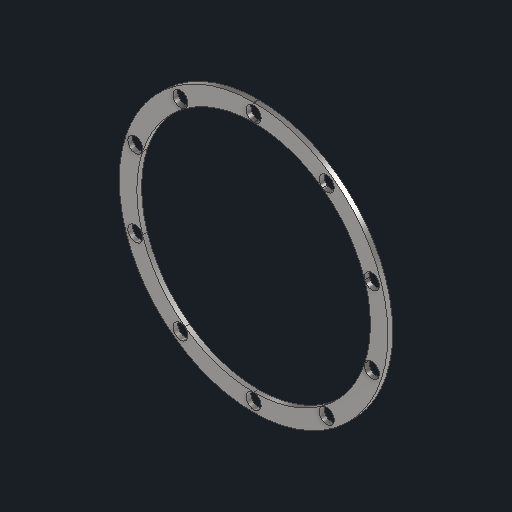
# Autodesk Inventor part: bracket 1
Saved by Autodesk Inventor 2023 (Build 270158000, 158)
## iProperties
Created: 2022-07-21
Part Number: bracket 1
Material: Stainless Steel
Document SubType Name: Modeling
Designer: station
Density: 8 g/cm^3
Appearance: Semi-Polished
Mass: 114.58 g
Surface Area: 134.314 cm^2
Volume: 14.3225 cm^3
Author: station
Autodesk Inventor part; units mm, degrees
ref_plane "YZ Plane" through (0, 0, 0) normal (1, 0, 0) x (0, 1, 0)
ref_plane "XZ Plane" through (0, 0, 0) normal (0, 1, 0) x (-1, 0, 0)
ref_plane "XY Plane" through (0, 0, 0) normal (0, 0, 1) x (1, 0, 0)
sketch "Sketch1" plane through (0, 0, 0) normal (0, 0, 1) x (1, 0, 0)
  point P0 (0, 0)
sketch "Sketch2" plane through (0, 0, 0) normal (0, 0, 1) x (1, 0, 0)
  circle A0 centre (0, 0) radius 73.505
  circle A1 centre (0, 0) radius 84.555
  line L0 (0, 0) -> (0, 267.2238)
  line L1 (0, 73.505) -> (0, 78.2675)
  circle A2 centre (0, 78.2675) radius 4.7625
  circle A3 centre (-46.0045, 63.3197) radius 4.7625
  circle A4 centre (-74.4368, 24.186) radius 4.7625
  circle A5 centre (-74.4368, -24.186) radius 4.7625
  circle A6 centre (-46.0045, -63.3197) radius 4.7625
  circle A7 centre (0, -78.2675) radius 4.7625
  circle A8 centre (46.0045, -63.3197) radius 4.7625
  circle A9 centre (74.4368, -24.186) radius 4.7625
  circle A10 centre (74.4368, 24.186) radius 4.7625
  circle A11 centre (46.0045, 63.3197) radius 4.7625
  point P0 (0, 73.505)
  point P1 (43.2052, 59.4668)
  point P2 (69.9074, 22.7143)
  point P3 (69.9074, -22.7143)
  point P4 (43.2052, -59.4668)
  point P5 (0, -73.505)
  point P6 (-43.2052, -59.4668)
  point P7 (-69.9074, -22.7143)
  point P8 (-69.9074, 22.7143)
  point P9 (-43.2052, 59.4668)
  dimension "d0" = 147.01
  dimension "d1" = 169.11
  dimension "d3" = 4.7625
  dimension "d4" = 9.525
  dimension "d7" = 360
  constraints: 11 centre point, 4 end point, 3 coincident, 2 point on line, 1 vertical, 24 other
  measures "d1" diameter of A1
  measures "d3" distance of L1.start L1.end
  measures "d4" diameter of A2
extrude "Extrusion1" add sketch "Sketch2" along normal blind 3
sketch "Sketch3" plane through (0, 0, 3) normal (0, 0, 1) x (1, 0, 0)
  circle A0 centre (0, 0) radius 84.555 projected
  line L0 (0, 84.555) -> (0, 84.055)
  line L1 (0.25, 83.8031) -> (-0.25, 83.8031)
  line L2 (-0.25, 83.8031) -> (-0.25, 84.3031)
  line L3 (-0.25, 84.3031) -> (0.25, 84.3031)
  line L4 (0.25, 84.3031) -> (0.25, 83.8031)
  line L5 (0.25, 83.8031) -> (-0.25, 84.3031) construction
  line L6 (-0.25, 83.8031) -> (0.25, 84.3031) construction
  point P0 (0, 84.0531)
  dimension "d11" = 0.5
  dimension "d15" = 0.5
  dimension "d16" = 0.5
  constraints: 14 end point, 2 midpoint, 2 parallel, 1 horizontal, 1 perpendicular, 1 point on line, 1 vertical, 1 vertical alignment, 1 other
  measures "d11" distance of L0.start L0.end
  measures "d15" distance of L2.end L3.end
  measures "d16" distance of L1.end L2.end
extrude "Extrusion2" cut sketch "Sketch3" against normal blind 10 contours L1 L2 L3 L4
body "Solid1"
